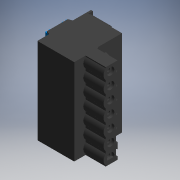
# Autodesk Inventor part: 4280684 14RD-1RR5.08-CLP-CBL
Saved by Autodesk Inventor 2017.3 (Build 213256000, 256)
## iProperties
Part Number: 4280684 14RD-1RR5.08-CLP-CBL
Material: Generic
Catalog Web Link: www.cadenas.de
Description: NEKM-C6 (p)-Terminal strip
Vendor: FESTO
Document SubType Name: Modeling
Designer: partserver
Manufacturer: FESTO
Mass: 12.0121 g
Surface Area: 60.2183 cm^2
Volume: 12.0121 cm^3
Density: 1 g/cm^3
Appearance: PSOLRGB-80-80-80
Category: PARTsolutions
Company: FESTO
Title: 4280684 14RD-1RR5.08-CLP-CBL
Author: Cadenas PARTsolutions
Comments: Terminal strip
PSOL_IDENT_0: {$CADENAS_DATA\23d-libs\festo\parts\n\nekm\parts\nekm_c6_parts.prj},201 {VTYP=3D},{NB=4280684 14RD-1
PSOL_IDENT_1: RR5.08-CLP-CBL},{LINA=4280684 14RD-1RR5.08-CLP-CBL},{NN=NEKM-C6 (p)},{DATE=16.05.2019 05:36:58},{GEO
PSOL_IDENT_2: MDATE=16.05.2019 05:36:56},{VERSION=},{LINEID=70},{WBVAR=},{WBNUMERIC=}  {NB=4280684 14RD-1RR5.08-CL
PSOL_IDENT_3: P-CBL},{LINA=4280684 14RD-1RR5.08-CLP-CBL},{KT=DUMMY},{TNR=4280684},{TYP=14RD-1RR5.08-CLP-CBL},{VERS=
PSOL_IDENT_4: 4},{N=7},{L=35.460},{L1=0.000}
NB: 4280684 14RD-1RR5.08-CLP-CBL
NN: NEKM-C6 (p)
NT: Terminal strip
NBSYN: $TNR. $TYP.
LINA: 4280684 14RD-1RR5.08-CLP-CBL
CATALOG: Festo
TNR: 4280684
TYP: 14RD-1RR5.08-CLP-CBL
VERS: 4
N: 7
L: 35.46
L1: 0
SUPPLIER: FESTO
ARTICLENO: 4280684 14RD-1RR5.08-CLP-CBL
BOMINFO: 4280684 14RD-1RR5.08-CLP-CBL
CREATOR: CADENAS GmbH
Autodesk Inventor part; units mm, degrees
ref_plane "YZ Plane" through (0, 0, 0) normal (1, 0, 0) x (0, 1, 0)
ref_plane "XZ Plane" through (0, 0, 0) normal (0, 1, 0) x (-1, 0, 0)
ref_plane "XY Plane" through (0, 0, 0) normal (0, 0, 1) x (1, 0, 0)
sketch "Sketch_1" plane through (0, 0, 0) normal (0, 0, 1) x (1, 0, 0)
  line L0 (-0.5, -11.05) -> (14.5, -11.05)
  arc A0 (14.5, -11.05) -> (14.7, -10.85) centre (14.5, -10.85) ccw
  line L1 (14.7, -10.85) -> (14.7, -6.4148)
  arc A1 (14.8974, -6.1329) -> (14.7, -6.4148) centre (15, -6.4148) ccw
  line L2 (14.8974, -6.1329) -> (16.0026, -5.7306)
  arc A2 (16.0026, -5.7306) -> (16.2, -5.4487) centre (15.9, -5.4487) ccw
  line L3 (16.2, -5.4487) -> (16.2, 2.7887)
  arc A3 (16.2, 2.7887) -> (16.0026, 3.0706) centre (15.9, 2.7887) ccw
  line L4 (16.0026, 3.0706) -> (14.8974, 3.4729)
  arc A4 (14.7, 3.7548) -> (14.8974, 3.4729) centre (15, 3.7548) ccw
  line L5 (14.7, 3.7548) -> (14.7, 10.85)
  arc A5 (14.7, 10.85) -> (14.5, 11.05) centre (14.5, 10.85) ccw
  line L6 (14.5, 11.05) -> (13.9, 11.05)
  line L7 (13.9, 11.05) -> (13.9, 9.15)
  line L8 (13.9, 9.15) -> (0, 9.15)
  line L9 (0, 9.15) -> (0, -0.584)
  line L10 (0, -0.584) -> (-0.5, -1.45)
  line L11 (-0.5, -1.45) -> (-0.5, -11.05)
  constraints: 24 end point, 12 point on circle, 6 centre point
extrude "Extrusion1" add sketch "Sketch_1" along normal mid plane 35.46
sketch "Sketch_2" plane through (14.7, 0, 0) normal (1, 0, 0) x (0, 0, -1)
  line L0 (-17.29, 3.755) -> (-17.29, 1.095)
  line L1 (-17.29, 1.095) -> (-13.19, 1.095)
  line L2 (-13.19, 1.095) -> (-13.19, 3.755)
  line L3 (-13.19, 3.755) -> (-17.29, 3.755)
  constraints: 8 end point
extrude "Extrusion2" cut sketch "Sketch_2" along normal blind 1.5
pattern_linear "Rectangular Pattern1" count 7 spacing 5.08 along (0, 0, -1) count 2 spacing 7.51 along (0, -1, 0) of "Extrusion2"
sketch "Sketch_4" plane through (0, 0, 17.19) normal (0, 0, 1) x (1, 0, 0)
  line L0 (14.7, 1.095) -> (16.7, 1.095)
  arc A0 (16.7, 1.095) -> (16.9, 1.295) centre (16.7, 1.295) ccw
  line L1 (16.9, 1.295) -> (16.9, 1.4099)
  arc A1 (16.9, 1.4099) -> (16.7041, 1.654) centre (16.65, 1.4099) ccw
  line L2 (16.7041, 1.654) -> (16.0359, 1.8021)
  arc A2 (16.0359, 2.3879) -> (16.0359, 1.8021) centre (16.1008, 2.095) ccw
  line L3 (16.0359, 2.3879) -> (16.7041, 2.536)
  arc A3 (16.7041, 2.536) -> (16.9, 2.7801) centre (16.65, 2.7801) ccw
  line L4 (16.9, 2.7801) -> (16.9, 2.895)
  arc A4 (16.9, 2.895) -> (16.7, 3.095) centre (16.7, 2.895) ccw
  line L5 (16.7, 3.095) -> (14.7, 3.095)
  line L6 (14.7, 3.095) -> (14.7, 1.095)
  constraints: 14 end point, 10 point on circle, 5 centre point
extrude "Extrusion3" add sketch "Sketch_4" against normal blind 3.9
pattern_linear "Rectangular Pattern2" count 7 spacing 5.08 along (0, 0, -1) count 2 spacing 6.85 along (0, -1, 0) of "Extrusion3"
sketch "Sketch_6" plane through (14.7, 0, 0) normal (1, 0, 0) x (0, 0, -1)
  arc A0 (-17.34, 4.6388) -> (-16.3455, 3.695) centre (-15.44, 5.645) ccw
  line L0 (-16.3455, 3.695) -> (-14.5345, 3.695)
  arc A1 (-14.5345, 3.695) -> (-14.5345, 7.595) centre (-15.44, 5.645) ccw
  line L1 (-14.5345, 7.595) -> (-16.3455, 7.595)
  arc A2 (-16.3455, 7.595) -> (-17.34, 6.6512) centre (-15.44, 5.645) ccw
  line L2 (-17.34, 6.6512) -> (-17.34, 4.6388)
  constraints: 6 end point, 6 point on circle, 3 centre point
extrude "Extrusion4" cut sketch "Sketch_6" against normal blind 3.85
pattern_linear "Rectangular Pattern3" count 2 spacing 13.95 along (0, -1, 0) of "Extrusion4"
sketch "Sketch_8" plane through (14.7, 0, 0) normal (1, 0, 0) x (0, 0, -1)
  arc A0 (-11.2655, 7.595) -> (-11.2655, 3.695) centre (-10.36, 5.645) ccw
  line L0 (-11.2655, 3.695) -> (-9.4545, 3.695)
  arc A1 (-9.4545, 3.695) -> (-9.4545, 7.595) centre (-10.36, 5.645) ccw
  line L1 (-9.4545, 7.595) -> (-11.2655, 7.595)
  constraints: 4 end point, 4 point on circle, 2 centre point
extrude "Extrusion5" cut sketch "Sketch_8" against normal blind 3.85
pattern_linear "Rectangular Pattern4" count 6 spacing 5.08 along (0, 0, -1) count 2 spacing 13.95 along (0, -1, 0) of "Extrusion5"
sketch "Sketch_10" plane through (13.9, 0, 0) normal (1, 0, 0) x (0, 0, -1)
  line L0 (-17.405, 9.15) -> (-12.875, 9.15)
  arc A0 (-12.875, 9.15) -> (-17.405, 9.15) centre (-15.14, 8.75) ccw
  constraints: 2 end point, 2 point on circle, 1 centre point
extrude "Extrusion6" add sketch "Sketch_10" against normal blind 9.7
sketch "Pattern_5_SKETCH_1" plane through (13.9, 0, 0) normal (1, 0, 0) x (0, 0, -1)
  line L0 (-12.425, 9.15) -> (-7.895, 9.15)
  arc A0 (-7.895, 9.15) -> (-12.425, 9.15) centre (-10.16, 8.75) ccw
  constraints: 2 end point, 2 point on circle, 1 centre point
sketch "Pattern_5_SKETCH_2" plane through (13.9, 0, 0) normal (1, 0, 0) x (0, 0, -1)
  line L0 (-7.345, 9.15) -> (-2.815, 9.15)
  arc A0 (-2.815, 9.15) -> (-7.345, 9.15) centre (-5.08, 8.75) ccw
  constraints: 2 end point, 2 point on circle, 1 centre point
sketch "Pattern_5_SKETCH_3" plane through (13.9, 0, 0) normal (1, 0, 0) x (0, 0, -1)
  line L0 (-2.265, 9.15) -> (2.265, 9.15)
  arc A0 (2.265, 9.15) -> (-2.265, 9.15) centre (0, 8.75) ccw
  constraints: 2 end point, 2 point on circle, 1 centre point
sketch "Pattern_5_SKETCH_4" plane through (13.9, 0, 0) normal (1, 0, 0) x (0, 0, -1)
  line L0 (2.815, 9.15) -> (7.345, 9.15)
  arc A0 (7.345, 9.15) -> (2.815, 9.15) centre (5.08, 8.75) ccw
  constraints: 2 end point, 2 point on circle, 1 centre point
sketch "Pattern_5_SKETCH_5" plane through (13.9, 0, 0) normal (1, 0, 0) x (0, 0, -1)
  line L0 (7.895, 9.15) -> (12.425, 9.15)
  arc A0 (12.425, 9.15) -> (7.895, 9.15) centre (10.16, 8.75) ccw
  constraints: 2 end point, 2 point on circle, 1 centre point
sketch "Pattern_5_SKETCH_6" plane through (13.9, 0, 0) normal (1, 0, 0) x (0, 0, -1)
  line L0 (12.975, 9.15) -> (17.505, 9.15)
  arc A0 (17.505, 9.15) -> (12.975, 9.15) centre (15.24, 8.75) ccw
  constraints: 2 end point, 2 point on circle, 1 centre point
extrude "Extrusion7" add sketch "Pattern_5_SKETCH_1" against normal blind 9.7
extrude "Extrusion8" add sketch "Pattern_5_SKETCH_2" against normal blind 9.7
extrude "Extrusion9" add sketch "Pattern_5_SKETCH_3" against normal blind 9.7
extrude "Extrusion10" add sketch "Pattern_5_SKETCH_4" against normal blind 9.7
extrude "Extrusion11" add sketch "Pattern_5_SKETCH_5" against normal blind 9.7
extrude "Extrusion12" add sketch "Pattern_5_SKETCH_6" against normal blind 9.7
sketch "Sketch_12" plane through (0, 0, 0) normal (0, 0, 1) x (1, 0, 0)
  line L0 (2, 11.05) -> (2, 9.15)
  line L1 (2, 9.15) -> (4.2, 9.15)
  line L2 (4.2, 9.15) -> (6.1, 11.05)
  line L3 (6.1, 11.05) -> (2, 11.05)
  constraints: 8 end point
extrude "Extrusion13" cut sketch "Sketch_12" along normal mid plane 35.46
sketch "Sketch_13" plane through (14.7, 0, 0) normal (1, 0, 0) x (0, 0, -1)
  line L0 (-16.39, 9.305) -> (-16.39, 8.155)
  line L1 (-16.39, 8.155) -> (-14.09, 8.155)
  line L2 (-14.09, 8.155) -> (-14.09, 9.305)
  arc A0 (-14.09, 9.305) -> (-16.39, 9.305) centre (-15.24, 9.305) ccw
  constraints: 6 end point, 2 point on circle, 1 centre point
extrude "Extrusion14" cut sketch "Sketch_13" against normal blind 9.35
pattern_linear "Rectangular Pattern5" count 7 spacing 5.08 along (0, 0, -1) of "Extrusion14"
sketch "Sketch_15" plane through (0, 11.05, 0) normal (0, 1, 0) x (1, 0, 0)
  arc A0 (5.35, -14.09) -> (5.35, -16.39) centre (5.35, -15.24) ccw
  line L0 (5.35, -16.39) -> (6.5, -16.39)
  line L1 (6.5, -16.39) -> (6.5, -14.09)
  line L2 (6.5, -14.09) -> (5.35, -14.09)
  constraints: 6 end point, 2 point on circle, 1 centre point
extrude "Extrusion15" cut sketch "Sketch_15" against normal blind 2.895
pattern_linear "Rectangular Pattern6" count 7 spacing 5.08 along (0, 0, -1) of "Extrusion15"
sketch "Sketch_17" plane through (-0.5, 0, 0) normal (1, 0, 0) x (0, 0, -1)
  line L0 (-17.73, -6.35) -> (-17.34, -6.35)
  arc A0 (-17.34, -6.35) -> (-13.14, -6.35) centre (-15.24, -4.35) ccw
  line L1 (-13.14, -6.35) -> (-12.26, -6.35)
  arc A1 (-12.26, -6.35) -> (-8.06, -6.35) centre (-10.16, -4.35) ccw
  line L2 (-8.06, -6.35) -> (-7.18, -6.35)
  arc A2 (-7.18, -6.35) -> (-2.98, -6.35) centre (-5.08, -4.35) ccw
  line L3 (-2.98, -6.35) -> (-2.1, -6.35)
  arc A3 (-2.1, -6.35) -> (2.1, -6.35) centre (0, -4.35) ccw
  line L4 (2.1, -6.35) -> (2.98, -6.35)
  arc A4 (2.98, -6.35) -> (7.18, -6.35) centre (5.08, -4.35) ccw
  line L5 (7.18, -6.35) -> (8.06, -6.35)
  arc A5 (8.06, -6.35) -> (12.26, -6.35) centre (10.16, -4.35) ccw
  line L6 (12.26, -6.35) -> (13.14, -6.35)
  arc A6 (13.14, -6.35) -> (17.34, -6.35) centre (15.24, -4.35) ccw
  line L7 (17.34, -6.35) -> (17.73, -6.35)
  line L8 (17.73, -6.35) -> (17.73, -1.45)
  line L9 (17.73, -1.45) -> (16.5, -1.45)
  line L10 (16.5, -1.45) -> (16.8926, -2.13)
  line L11 (16.8926, -2.13) -> (13.5874, -2.13)
  line L12 (13.5874, -2.13) -> (13.98, -1.45)
  line L13 (13.98, -1.45) -> (11.42, -1.45)
  line L14 (11.42, -1.45) -> (11.8126, -2.13)
  line L15 (11.8126, -2.13) -> (8.5074, -2.13)
  line L16 (8.5074, -2.13) -> (8.9, -1.45)
  line L17 (8.9, -1.45) -> (6.34, -1.45)
  line L18 (6.34, -1.45) -> (6.7326, -2.13)
  line L19 (6.7326, -2.13) -> (3.4274, -2.13)
  line L20 (3.4274, -2.13) -> (3.82, -1.45)
  line L21 (3.82, -1.45) -> (1.26, -1.45)
  line L22 (1.26, -1.45) -> (1.6526, -2.13)
  line L23 (1.6526, -2.13) -> (-1.6526, -2.13)
  line L24 (-1.6526, -2.13) -> (-1.26, -1.45)
  line L25 (-1.26, -1.45) -> (-3.82, -1.45)
  line L26 (-3.82, -1.45) -> (-3.4274, -2.13)
  line L27 (-3.4274, -2.13) -> (-6.7326, -2.13)
  line L28 (-6.7326, -2.13) -> (-6.34, -1.45)
  line L29 (-6.34, -1.45) -> (-8.9, -1.45)
  line L30 (-8.9, -1.45) -> (-8.5074, -2.13)
  line L31 (-8.5074, -2.13) -> (-11.8126, -2.13)
  line L32 (-11.8126, -2.13) -> (-11.42, -1.45)
  line L33 (-11.42, -1.45) -> (-13.98, -1.45)
  line L34 (-13.98, -1.45) -> (-13.5874, -2.13)
  line L35 (-13.5874, -2.13) -> (-16.8926, -2.13)
  line L36 (-16.8926, -2.13) -> (-16.5, -1.45)
  line L37 (-16.5, -1.45) -> (-17.73, -1.45)
  line L38 (-17.73, -1.45) -> (-17.73, -6.35)
  constraints: 78 end point, 14 point on circle, 7 centre point
extrude "Extrusion16" add sketch "Sketch_17" against normal blind 8.3
sketch "Sketch17" plane through (-8.8, 0, 0) normal (-1, 0, 0) x (0, 0, 1)
  point P0 (15.24, -4.35)
hole "Hole1" at (-8.8, -4.35, 15.24) direction (1, 0, 0) diameter 1.4 depth 2 counterbore diameter 3 counterbore depth 1
pattern_linear "Rectangular Pattern7" count 7 spacing 5.08 along (0, 0, -1) of "Hole1"
sketch "Sketch_20" plane through (0, -4.35, 0) normal (0, 1, 0) x (1, 0, 0)
  line L0 (-8.8, -16.94) -> (-7.8, -16.94)
  line L1 (-7.8, -16.94) -> (-7.8, -15.94)
  line L2 (-7.8, -15.94) -> (-8.8, -15.94)
  line L3 (-8.8, -15.94) -> (-8.8, -16.94)
  constraints: 8 end point
extrude "Extrusion17" add sketch "Sketch_20" along normal mid plane 4
sketch "Sketch_21" plane through (0, 0, 14.3) normal (0, 0, 1) x (1, 0, 0)
  arc A0 (-4.9014, 0.6066) -> (-4.86, 0.292) centre (-4.76, 0.4652) ccw
  line L0 (-4.86, 0.292) -> (-4.1642, -0.1097)
  arc A1 (-4.1642, -0.1097) -> (-3.8021, -0.0621) centre (-4.0142, 0.1501) ccw
  line L1 (-3.8021, -0.0621) -> (-3.53, 0.21)
  line L2 (-3.53, 0.21) -> (-0.3256, 0.3499)
  arc A2 (-0.3, -0.249) -> (-0.3256, 0.3499) centre (-0.3, 0.051) ccw
  arc A3 (-0.3, -0.249) -> (-0.5, -0.449) centre (-0.3, -0.449) ccw
  line L3 (-0.5, -0.449) -> (-0.5, -2.76)
  line L4 (-0.5, -2.76) -> (0.5, -2.76)
  line L5 (0.5, -2.76) -> (0.5, 2.6984)
  line L6 (0.5, 2.6984) -> (0, 2.6984)
  arc A4 (-0.2325, 2.4061) -> (0, 2.6984) centre (-0.3, 2.6984) ccw
  line L7 (-0.2325, 2.4061) -> (-3.7536, 1.5932)
  arc A5 (-3.7536, 1.5932) -> (-4.1152, 1.3928) centre (-3.5849, 0.8624) ccw
  line L8 (-4.1152, 1.3928) -> (-4.9014, 0.6066)
  constraints: 18 end point, 12 point on circle, 6 centre point
extrude "Extrusion18" add sketch "Sketch_21" against normal blind 1.6
sketch "Sketch_22" plane through (0, 0, -14.3) normal (0, 0, 1) x (1, 0, 0)
  arc A0 (-4.9014, 0.6066) -> (-4.86, 0.292) centre (-4.76, 0.4652) ccw
  line L0 (-4.86, 0.292) -> (-4.1642, -0.1097)
  arc A1 (-4.1642, -0.1097) -> (-3.8021, -0.0621) centre (-4.0142, 0.1501) ccw
  line L1 (-3.8021, -0.0621) -> (-3.53, 0.21)
  line L2 (-3.53, 0.21) -> (-0.3256, 0.3499)
  arc A2 (-0.3, -0.249) -> (-0.3256, 0.3499) centre (-0.3, 0.051) ccw
  arc A3 (-0.3, -0.249) -> (-0.5, -0.449) centre (-0.3, -0.449) ccw
  line L3 (-0.5, -0.449) -> (-0.5, -2.76)
  line L4 (-0.5, -2.76) -> (0.5, -2.76)
  line L5 (0.5, -2.76) -> (0.5, 2.6984)
  line L6 (0.5, 2.6984) -> (0, 2.6984)
  arc A4 (-0.2325, 2.4061) -> (0, 2.6984) centre (-0.3, 2.6984) ccw
  line L7 (-0.2325, 2.4061) -> (-3.7536, 1.5932)
  arc A5 (-3.7536, 1.5932) -> (-4.1152, 1.3928) centre (-3.5849, 0.8624) ccw
  line L8 (-4.1152, 1.3928) -> (-4.9014, 0.6066)
  constraints: 18 end point, 12 point on circle, 6 centre point
extrude "Extrusion19" add sketch "Sketch_22" along normal blind 1.6
ref_plane "ANBAU_XY" through (0, 0, 0) normal (0, 1, 0) x (1, 0, 0)
ref_plane "ANBAU_YZ" through (0, 0, 0) normal (1, 0, 0) x (0, 0, -1)
ref_plane "ANBAU_ZX" through (0, 0, 0) normal (0, 0, -1) x (0, 1, 0)
body "Solid1"
